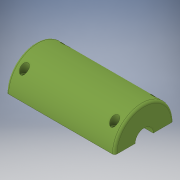
# Autodesk Inventor part: Slider Mount_C
Saved by Autodesk Inventor 2018 (Build 220112000, 112)
## iProperties
Created: 2018-01-08
Part Number: Slider Mount_C
Material: ABS Plastic
Document SubType Name: Modeling
Designer: njcfu
Density: 1.06 g/cm^3
Appearance: Olive Green
Author: njcfu
Autodesk Inventor part; units mm, degrees
ref_plane "YZ Plane" through (0, 0, 0) normal (1, 0, 0) x (0, 1, 0)
ref_plane "XY Plane" through (0, 0, 0) normal (0, 0, 1) x (1, 0, 0)
sketch "Sketch1" plane through (0, 0, 0) normal (1, 0, 0) x (0, 1, 0)
  arc A0 (0, -25.4) -> (0, 25.4) centre (0, 0) ccw
  arc A1 (0, -41.275) -> (0, 41.275) centre (0, 0) ccw
  line L0 (0, 41.275) -> (0, 25.4)
  line L1 (0, -25.4) -> (0, -41.275)
  dimension "d24" = 25.4
  dimension "d29" = 0
  dimension "d32" = 15.875
  dimension "d110" = 41.275
  constraints: 4 end point, 4 point on circle, 2 centre point, 2 coincident, 1 collinear, 1 vertical
  measures "d24" distance of A0.centre L0.end
  measures "d29" distance from line of point (0, 0) L1
  measures "d32" distance of L0.start L0.end
  measures "d110" radius of A1
extrude "Extrusion1" add sketch "Sketch1" along normal mid plane 49.9999
ref_plane "Work Plane2" through (0, 25.4, 0) normal (0, 1, 0) x (-1, 0, 0)
sketch "Sketch3" plane through (0, 25.4, 0) normal (0, 1, 0) x (-1, 0, 0)
  point P0 (0, 0)
sketch "Sketch4" plane through (0, 25.4, 0) normal (0, 1, 0) x (-1, 0, 0)
  line L0 (3.3655, 0.9525) -> (-3.3655, 0.9525)
  line L1 (-3.3655, 0.9525) -> (-3.3655, -0.9525)
  line L2 (-3.3655, -0.9525) -> (3.3655, -0.9525)
  line L3 (3.3655, -0.9525) -> (3.3655, 0.9525)
  line L4 (3.3655, 0.9525) -> (-3.3655, -0.9525) construction
  line L5 (-3.3655, 0.9525) -> (3.3655, -0.9525) construction
  point P0 (0, 0)
  dimension "d30" = 6.731
  dimension "d31" = 1.905
  constraints: 12 end point, 2 midpoint, 2 parallel, 1 horizontal, 1 perpendicular
  measures "d30" distance of L1.end L2.end
  measures "d31" distance of L2.end L0.start
extrude "Extrusion3" cut sketch "Sketch4" along normal blind 14.986 and the other way blind 1.27
sketch "Sketch5" plane through (-25, 0, 0) normal (-1, 0, 0) x (0, 0, 1)
  arc A0 (41.275, 0) -> (-41.275, 0) centre (0, 0) ccw
  arc A1 (25.4, 0) -> (-25.4, 0) centre (0, 0) ccw
  arc A2 (41.275, 0) -> (-41.275, 0) centre (0, 0) ccw projected
  line L0 (-41.275, 0) -> (-25.4, 0) projected
  line L1 (-41.275, 0) -> (-25.4, 0)
  line L2 (25.4, 0) -> (41.275, 0)
  dimension "d40" = 15.875
  constraints: 4 end point, 4 point on circle, 2 centre point, 2 coincident, 2 collinear
  measures "d40" distance of L2.start L2.end
extrude "Extrusion4" add sketch "Sketch5" along normal blind 12.7
sketch "Sketch6" plane through (25, 0, 0) normal (1, 0, 0) x (0, 0, -1)
  arc A0 (41.275, 0) -> (-41.275, 0) centre (0, 0) ccw
  arc A1 (25.4, 0) -> (-25.4, 0) centre (0, 0) ccw
  line L0 (-41.275, 0) -> (-25.4, 0)
  line L1 (25.4, 0) -> (41.275, 0)
  dimension "d44" = 25.4
  dimension "d45" = 15.875
  dimension "d46" = 15.875
  dimension "d111" = 41.275
  constraints: 4 end point, 4 point on circle, 2 centre point, 2 coincident, 2 horizontal
  measures "d44" radius of A1
  measures "d45" distance of L0.start L0.end
  measures "d46" distance of L1.start L1.end
  measures "d111" distance of L1.end point (0, 0)
extrude "Extrusion5" add sketch "Sketch6" along normal blind 12.7
sketch "Sketch7" plane through (-37.7, 0, 0) normal (-1, 0, 0) x (0, 0, 1)
  arc A0 (41.275, 0) -> (-41.275, 0) centre (0, 0) ccw
  arc A1 (12.7, 0) -> (-12.7, 0) centre (0, 0) ccw
  line L0 (-41.275, 0) -> (-12.7, 0)
  line L1 (12.7, 0) -> (41.275, 0)
  dimension "d50" = 12.7
  dimension "d51" = 28.575
  dimension "d112" = 41.275
  constraints: 4 end point, 4 point on circle, 2 centre point, 2 coincident, 2 point on line, 1 horizontal
  measures "d50" radius of A1
  measures "d51" distance of L0.start L0.end
  measures "d112" radius of A0
extrude "Extrusion6" add sketch "Sketch7" along normal blind 38.1
sketch "Sketch8" plane through (0, 0, 0) normal (1, 0, 0) x (0, 1, 0)
  line L0 (0, -12.7) -> (0, -25.4) projected
  arc A0 (0, -12.7) -> (0, 12.7) centre (0, 0) ccw projected
  line L1 (0, 0) -> (17.9605, 17.9605)
  line L2 (21.7705, 20.5005) -> (14.1505, 20.5005)
  line L3 (14.1505, 20.5005) -> (14.1505, 15.4205)
  line L4 (14.1505, 15.4205) -> (21.7705, 15.4205)
  line L5 (21.7705, 15.4205) -> (21.7705, 20.5005)
  arc A1 (0, -25.4) -> (0, 25.4) centre (0, 0) ccw projected
  dimension "d102" = 135
  dimension "d103" = 5.08
  dimension "d104" = 2.54
  dimension "d105" = 7.62
  dimension "d106" = 3.81
  constraints: 10 end point, 2 parallel, 1 coincident, 1 horizontal, 1 perpendicular, 1 point on circle
  measures "d102" angle of L0 L1
  measures "d103" distance of L2.end L3.end
  measures "d104" distance from line of L4 point (17.961, 17.961)
  measures "d105" distance of L2.start L2.end
  measures "d106" distance from line of point (17.961, 17.961) L5
extrude "Extrusion7" cut sketch "Sketch8" along normal mid plane 39.9999 contours A1 L2 L5 L4 | L4 L1 A1 | L4 L3 L2 A1 L1
sketch "Sketch9" plane through (37.7, 0, 0) normal (1, 0, 0) x (0, 0, -1)
  arc A0 (41.275, 0) -> (-41.275, 0) centre (0, 0) ccw
  arc A1 (12.7, 0) -> (-12.7, 0) centre (0, 0) ccw
  line L0 (-41.275, 0) -> (-12.7, 0)
  line L1 (12.7, 0) -> (41.275, 0)
  point P0 (0, 0)
  dimension "d68" = 12.7
  dimension "d69" = 28.575
  dimension "d70" = 12.7
  dimension "d71" = 41.275
  dimension "d113" = 41.275
  constraints: 4 end point, 4 point on circle, 2 centre point, 2 coincident, 2 point on line, 1 horizontal
  measures "d68" radius of A1
  measures "d69" distance of L0.start L0.end
  measures "d70" distance of L0.end point (0, 0)
  measures "d71" distance of L1.end point (0, 0)
  measures "d113" radius of A0
extrude "Extrusion8" add sketch "Sketch9" along normal blind 38.1
sketch "Sketch10" plane through (-37.7, 0, 12.7) normal (0, -1, 0) x (1, 0, 0)
  circle A0 centre (100.7999, 15.875) radius 2.413
  circle A1 centre (100.7999, -41.275) radius 2.413
  circle A2 centre (-25.4, -41.275) radius 2.413
  circle A3 centre (-25.4, 15.875) radius 2.413
  line L0 (113.4999, 28.575) -> (113.4999, 0) projected
  line L1 (-38.1, 28.575) -> (113.4999, 28.575) projected
  line L2 (-38.1, -53.975) -> (113.4999, -53.975) projected
  line L3 (113.4999, -25.4) -> (113.4999, -53.975) projected
  line L4 (-38.1, 0) -> (-38.1, 28.575) projected
  line L5 (-38.1, -53.975) -> (-38.1, -25.4) projected
  point P0 (37.7, -12.7)
  point P1 (12.7, 28.575)
  point P2 (12.7, -53.975)
  point P3 (0, 28.575)
  point P4 (0, -53.975)
  dimension "d74" = 4.826
  dimension "d75" = 12.7
  dimension "d76" = 12.7
  dimension "d77" = 12.7
  dimension "d78" = 12.7
  dimension "d79" = 4.826
  dimension "d80" = 12.7
  dimension "d81" = 12.7
  dimension "d82" = 12.7
  dimension "d83" = 12.7
  dimension "d84" = 4.826
  dimension "d85" = 4.826
  constraints: 4 centre point
  measures "d74" diameter of A0
  measures "d75" distance from line of L0 A0.centre
  measures "d76" distance from line of L1 A0.centre
  measures "d77" distance from line of L2 A1.centre
  measures "d78" distance from line of L3 A1.centre
  measures "d79" diameter of A1
  measures "d80" distance from line of L1 A3.centre
  measures "d81" distance from line of L4 A3.centre
  measures "d82" distance from line of L5 A2.centre
  measures "d83" distance from line of L2 A2.centre
  measures "d84" diameter of A2
  measures "d85" diameter of A3
extrude "Extrusion9" cut sketch "Sketch10" against normal blind 38.1
ref_plane "Work Plane3" through (-37.7, 28.4375, 12.7) normal (0, -1, 0) x (1, 0, 0)
sketch "Sketch11" plane through (-37.7, 28.4375, 12.7) normal (0, -1, 0) x (1, 0, 0)
  circle A0 centre (-25.4, 15.875) radius 5.08
  circle A1 centre (100.7999, 15.875) radius 5.0759
  circle A2 centre (100.7999, -41.275) radius 5.08
  circle A3 centre (-25.4, -41.275) radius 5.08
  circle A4 centre (-25.4, 15.875) radius 2.413 projected
  circle A5 centre (-25.4, -41.275) radius 2.413 projected
  circle A6 centre (100.7999, -41.275) radius 2.413 projected
  circle A7 centre (100.7999, 15.875) radius 2.413 projected
  point P0 (37.7, -12.7)
  dimension "d89" = 10.16
  dimension "d90" = 10.1518
  dimension "d91" = 10.16
  dimension "d92" = 10.16
  constraints: 4 centre point, 4 concentric
  measures "d89" diameter of A2
  measures "d90" diameter of A1
  measures "d91" diameter of A0
  measures "d92" diameter of A3
extrude "Extrusion10" cut sketch "Sketch11" along normal blind 7.62 and the other way blind 12.7
mirror "Mirror3" about plane through (0, 0, 0) normal (0, 0, 1) of "Extrusion7"
fillet "Fillet6" radius 3.175 2 edges at (-75.8, 41.275, 0) (75.8, 41.275, 0)
fillet "Fillet7" radius 0.254 4 edges at (0, 21.7705, 20.5005) (0, 21.7705, 15.4205) (0, 21.7705, -20.5005) (0, 21.7705, -15.4205)
body "Solid1"
